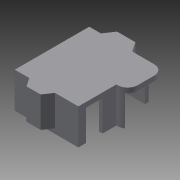
# Autodesk Inventor part: FelixOriginalTop
Saved by Autodesk Inventor 2015 SP1 (Build 190203100, 203)
## iProperties
Created: 2014-12-15
Part Number: FelixOriginalTop
Material: Generic
Document SubType Name: Modeling
Designer: Jack
Density: 1 g/cm^3
Appearance: Default
Author: Jack
Autodesk Inventor part; units mm, degrees
ref_plane "YZ Plane" through (0, 0, 0) normal (1, 0, 0) x (0, 1, 0)
ref_plane "XZ Plane" through (0, 0, 0) normal (0, 1, 0) x (-1, 0, 0)
ref_plane "XY Plane" through (0, 0, 0) normal (0, 0, 1) x (1, 0, 0)
sketch "Sketch1" plane through (0, 0, 0) normal (0, 0, 1) x (1, 0, 0)
  line L0 (0, 0) -> (0, 60.76)
  line L1 (51.9, 31.06) -> (51.9, 0)
  line L2 (51.9, 60.76) -> (61.1, 60.76)
  line L3 (61.1, 60.76) -> (61.1, 31.06)
  line L4 (61.1, 31.06) -> (51.9, 31.06)
  line L5 (9.5, 60.76) -> (14.8286, 68.66)
  line L6 (14.8286, 68.66) -> (29.7714, 68.66)
  line L7 (29.7714, 68.66) -> (35.1, 60.76)
  line L8 (11.8, 0) -> (16.5216, -7)
  line L9 (16.5216, -7) -> (28.0784, -7)
  line L10 (28.0784, -7) -> (32.8, 0)
  line L11 (22.3, 68.66) -> (22.3, -7) construction
  line L12 (0, 60.76) -> (9.5, 60.76)
  line L13 (35.1, 60.76) -> (51.9, 60.76)
  line L14 (0, 0) -> (11.8, 0)
  line L15 (32.8, 0) -> (51.9, 0)
  dimension "d0" = 51.9
  dimension "d1" = 60.76
  dimension "d2" = 9.2
  dimension "d3" = 29.7
  dimension "d11" = 25.6
  dimension "d12" = 21
  dimension "d13" = 29.6
  dimension "d14" = 124
  dimension "d15" = 124
  dimension "d16" = 124
  dimension "d17" = 124
  dimension "d18" = 7.9
  dimension "d19" = 7
  constraints: 32 end point, 6 perpendicular, 5 horizontal, 2 collinear, 2 horizontal alignment, 2 midpoint, 2 vertical, 1 point on line
  measures "d0" distance of L0.start L1.end
  measures "d1" distance of L0.start L0.end
  measures "d2" distance of L2.start L2.end
  measures "d3" distance between parallel lines of L4 L2
  measures "d11" distance of L7.end L5.start
  measures "d12" distance of L10.end L8.start
  measures "d13" distance between parallel lines of L1 L11
  measures "d14" angle of L13 L7
  measures "d15" angle of L5 L12
  measures "d16" angle of L8 L14
  measures "d17" angle of L10 L15
  measures "d18" distance between parallel lines of L13 L6
  measures "d19" distance between parallel lines of L15 L9
extrude "Extrusion1" add sketch "Sketch1" along normal blind 4
fillet "Fillet1" radius 8 2 edges at (61.1, 31.06, 2) (61.1, 60.76, 2)
sketch "Sketch2" plane through (0, 0, 0) normal (0, 0, -1) x (-1, 0, 0)
  line L0 (0, 0) -> (0, 60.76) projected
  line L1 (0, 60.76) -> (-9.5, 60.76) projected
  line L2 (-35.1, 60.76) -> (-53.1, 60.76) projected
  line L3 (0, 60.76) -> (0, 0) projected
  line L4 (0, 57.76) -> (-48.4, 57.76)
  line L5 (-48.4, 57.76) -> (-48.4, 60.76)
  line L6 (-35.1, 60.76) -> (-9.5, 60.76)
  dimension "d23" = 48.4
  dimension "d24" = 3
  constraints: 6 end point, 2 perpendicular, 2 point on line, 1 horizontal
  measures "d23" distance of L4.start L4.end
  measures "d24" distance of L4.end L5.end
extrude "Extrusion2" add sketch "Sketch2" along normal blind 25
sketch "Sketch3" plane through (0, 0, 0) normal (0, 0, -1) x (-1, 0, 0)
  line L0 (-35.1, 60.76) -> (-9.5, 60.76) projected
  line L1 (-9.5, 60.76) -> (-14.8286, 68.66) projected
  line L2 (-14.8286, 68.66) -> (-29.7714, 68.66) projected
  line L3 (-29.7714, 68.66) -> (-35.1, 60.76) projected
  point P0 (0, 0)
extrude "Extrusion3" add sketch "Sketch3" along normal blind 21
sketch "Sketch4" plane through (0, 0, 0) normal (0, 0, -1) x (-1, 0, 0)
  line L0 (-51.9, 31.06) -> (-51.9, 0) projected
  line L1 (-51.9, 0) -> (-32.8, 0) projected
  line L2 (-11.8, 0) -> (0, 0) projected
  line L3 (0, 0) -> (0, 57.76) projected
  line L4 (0, 3) -> (-48.9, 3)
  line L5 (-48.9, 3) -> (-48.9, 6.2)
  line L6 (-48.9, 6.2) -> (-51.9, 6.2)
  line L7 (-32.8, 0) -> (-11.8, 0)
  dimension "d29" = 3
  dimension "d30" = 3
  dimension "d31" = 3.2
  constraints: 8 end point, 2 horizontal, 2 perpendicular, 2 point on line
  measures "d29" distance of L5.end L6.end
  measures "d30" distance between parallel lines of L2 L4
  measures "d31" distance between parallel lines of L4 L6
extrude "Extrusion4" add sketch "Sketch4" along normal blind 25
sketch "Sketch5" plane through (0, 0, 0) normal (0, 0, -1) x (-1, 0, 0)
  line L0 (-11.8, 0) -> (-32.8, 0) projected
  line L1 (-32.8, 0) -> (-28.0784, -7) projected
  line L2 (-28.0784, -7) -> (-16.5216, -7) projected
  line L3 (-16.5216, -7) -> (-11.8, 0) projected
  point P0 (0, 0)
extrude "Extrusion5" add sketch "Sketch5" along normal blind 21
sketch "Sketch6" plane through (0, 0, 0) normal (0, 0, -1) x (-1, 0, 0)
  line L0 (-48.9, 3) -> (0, 3) projected
  line L1 (0, 3) -> (0, 57.76) projected
  line L2 (0, 57.76) -> (-48.4, 57.76) projected
  line L3 (-3, 3) -> (-3, 57.76)
  point P0 (0, 0)
  dimension "d36" = 3
  constraints: 2 end point, 2 point on line, 1 perpendicular
  measures "d36" distance between parallel lines of L1 L3
extrude "Extrusion6" add sketch "Sketch6" along normal blind 20.4
sketch "Sketch7" plane through (0, 0, 0) normal (0, 0, -1) x (-1, 0, 0)
  line L0 (-48.4, 60.76) -> (-53.1, 60.76) projected
  arc A0 (-61.1, 39.06) -> (-53.1, 31.06) centre (-53.1, 39.06) ccw projected
  line L1 (-53.1, 31.06) -> (-51.9, 31.06) projected
  line L2 (-51.9, 31.06) -> (-51.9, 6.2) projected
  line L3 (-51.9, 6.2) -> (-48.9, 6.2) projected
  line L4 (-51.9, 0) -> (-51.9, 31.06) projected
  line L5 (-51.9, 19.7) -> (-48.9, 19.7)
  line L6 (-48.9, 19.7) -> (-48.9, 34.06)
  line L7 (-48.9, 34.06) -> (-53.1, 34.06)
  arc A1 (-54.8897, 34.3913) -> (-53.1, 34.06) centre (-53.1, 39.06) ccw
  line L8 (-54.8897, 34.3913) -> (-57.5322, 32.4)
  arc A2 (-61.1, 39.06) -> (-53.1, 31.06) centre (-53.1, 39.06) ccw projected
  point P0 (0, 0)
  dimension "d39" = 3
  dimension "d40" = 3
  dimension "d41" = 13.5
  dimension "d42" = 37
  dimension "d43" = 12.7
  constraints: 8 end point, 4 point on circle, 3 perpendicular, 1 centre point, 1 coincident, 1 point on line, 1 tangent
  measures "d39" radial gap between concentric circles of A0 A1
  measures "d40" distance between parallel lines of L2 L6
  measures "d41" distance between parallel lines of L3 L5
  measures "d42" angle of L0 L8
  measures "d43" vertical distance of L5.start L8.end
extrude "Extrusion7" add sketch "Sketch7" along normal blind 25
body "Solid1"
